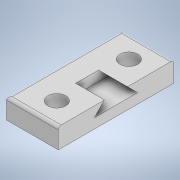
# Autodesk Inventor part: Dovetail_holder_V2
Saved by Autodesk Inventor 2020 (Build 240168000, 168)
## iProperties
Created: 2020-11-04
Part Number: Dovetail_holder_V2
Material: Generic
Document SubType Name: Modeling
Designer: Allesfresser
Density: 1 g/cm^3
Appearance: Default
Author: Allesfresser
Autodesk Inventor part; units mm, degrees
ref_plane "YZ Plane" through (0, 0, 0) normal (1, 0, 0) x (0, 1, 0)
ref_plane "XZ Plane" through (0, 0, 0) normal (0, 1, 0) x (-1, 0, 0)
ref_plane "XY Plane" through (0, 0, 0) normal (0, 0, 1) x (1, 0, 0)
sketch "Sketch1" plane through (0, 0, 0) normal (0, 1, 0) x (-1, 0, 0)
  line L0 (-9, 20) -> (9, 20)
  line L1 (9, 20) -> (9, -20)
  line L2 (9, -20) -> (-9, -20)
  line L3 (-9, -20) -> (-9, 20)
  line L4 (-9, 20) -> (9, -20) construction
  line L5 (9, 20) -> (-9, -20) construction
  point P0 (0, 0)
  dimension "d0" = 18
  dimension "d1" = 40
  constraints: 12 end point, 2 midpoint, 2 parallel, 1 horizontal, 1 perpendicular
  measures "d0" distance of L1.end L2.end
  measures "d1" distance of L0.end L1.end
extrude "Extrusion1" add sketch "Sketch1" along normal blind 7
sketch "Sketch2" plane through (0, 7, 0) normal (0, 1, 0) x (1, 0, 0)
  circle A0 centre (1, -12.5) radius 3.1
  line L0 (-9, -20) -> (9, -20) projected
  line L1 (9, -20) -> (9, 20) projected
  point P0 (0, 0)
  dimension "d4" = 6.2
  dimension "d5" = 7.5
  dimension "d6" = 8
  constraints: 1 centre point
  measures "d4" diameter of A0
  measures "d5" distance from line of L0 A0.centre
  measures "d6" distance from line of L1 A0.centre
extrude "Extrusion2" cut sketch "Sketch2" against normal through all
mirror "Mirror1" about plane through (0, 0, 0) normal (0, 0, 1) of "Extrusion2"
sketch "Sketch3" plane through (9, 0, 20) normal (1, 0, 0) x (0, 0, -1)
  line L0 (0, 7) -> (40, 7) projected
  line L1 (16, 7) -> (12.4645, 3.4645)
  line L2 (16, 7) -> (21, 7) construction
  line L3 (16, 7) -> (24, 7)
  line L4 (16, 7) -> (24, 7) construction
  line L5 (24, 7) -> (27.5355, 3.4645)
  line L6 (27.5355, 3.4645) -> (12.4645, 3.4645)
  point P0 (20, 0)
  dimension "d9" = 5
  dimension "d10" = 135
  dimension "d11" = 16
  dimension "d12" = 8
  dimension "d13" = 0
  dimension "d14" = 5
  dimension "d15" = 135
  constraints: 12 end point, 2 equal length, 2 horizontal, 2 point on line, 1 collinear, 1 parallel
  measures "d9" distance of L1.start L1.end
  measures "d10" angle of L1 L2
  measures "d11" distance of L0.start L1.start
  measures "d12" distance of L1.start L3.end
  measures "d13" distance between parallel lines of L3 L4
  measures "d14" distance of L3.end L5.end
  measures "d15" angle of L3 L5
extrude "Extrusion3" cut sketch "Sketch3" against normal blind 10
fillet "Fillet1" radius 1 3 edges at (0, 7, -20) (-9, 7, 0) (0, 7, 20)
body "Solid1"
